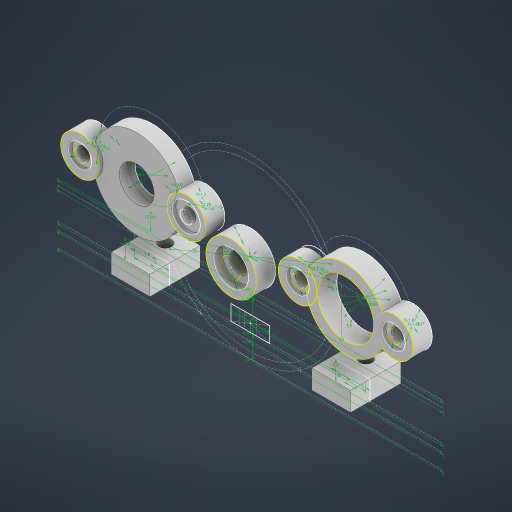
# Autodesk Inventor part: Motormount
Saved by Autodesk Inventor 2023.5 (Build 275446000, 446)
## iProperties
Created: 2024-12-07
Part Number: Motormount
Material: 一般
Document SubType Name: Modeling
Designer: IshiiLabHonda
Density: 1 g/cm^3
Appearance: 既定
Author: IshiiLabHonda
Autodesk Inventor part; units mm, degrees
ref_plane "YZ Plane" through (0, 0, 0) normal (1, 0, 0) x (0, 1, 0)
ref_plane "XZ Plane" through (0, 0, 0) normal (0, 1, 0) x (-1, 0, 0)
ref_plane "XY Plane" through (0, 0, 0) normal (0, 0, 1) x (1, 0, 0)
sketch "blueprint" plane through (0, 0, 0) normal (0, 0, 1) x (1, 0, 0)
  line L0 (0, 0) -> (0, 1) construction
  line L1 (0, 0) -> (1, 0) construction
  circle A0 centre (0, 0) radius 1.25
  circle A1 centre (0, 0) radius 11.5 construction
  line L2 (-25, -11.5) -> (25, -11.5) construction
  line L3 (-25, -9.5) -> (25, -9.5) construction
  line L4 (-25, -8.5) -> (25, -8.5) construction
  line L5 (-25, -4.5) -> (25, -4.5) construction
  circle A2 centre (0, 0) radius 10.65 construction
  circle A3 centre (-12.6949, 2.8) radius 2.25
  circle A4 centre (14.8381, 2.8) radius 4.35 construction
  circle A5 centre (14.8381, 2.8) radius 3.6 construction
  line L6 (-25, -3.7) -> (25, -3.7) construction
  circle A6 centre (-12.6949, 2.8) radius 4.26 construction
  circle A7 centre (-19.5799, 2.8) radius 0.625 construction
  circle A8 centre (-5.8099, 2.8) radius 0.625 construction
  circle A9 centre (-12.6949, 2.8) radius 6.885 construction
  circle A10 centre (-19.5799, 2.8) radius 1.825 construction
  circle A11 centre (-5.8099, 2.8) radius 1.825 construction
  circle A12 centre (14.8381, 2.8) radius 5.1
  circle A13 centre (14.8381, 2.8) radius 6.225 construction
  circle A14 centre (21.0631, 2.8) radius 0.625 construction
  circle A15 centre (8.6131, 2.8) radius 0.625 construction
  circle A16 centre (21.0631, 2.8) radius 1.825 construction
  circle A17 centre (-19.5799, 2.8) radius 0.8
  circle A18 centre (-5.8099, 2.8) radius 0.8
  circle A19 centre (21.0631, 2.8) radius 0.8
  circle A20 centre (-19.5799, 2.8) radius 2.5
  circle A21 centre (-5.8099, 2.8) radius 2.5
  circle A22 centre (21.0631, 2.8) radius 2.5
  circle A23 centre (14.8381, 2.8) radius 3.65
  circle A24 centre (0, 0) radius 3.25
  line L7 (-15, -4.5) -> (-15, -8.5) construction
  line L8 (15, -4.5) -> (15, -8.5) construction
  line L9 (-10.5, -8.5) -> (-10.5, -6)
  line L10 (-15.5, -8.5) -> (-15.5, -6)
  line L11 (-15.5, -6) -> (-10.5, -6)
  line L12 (-13, -6) -> (-13, -8.5)
  line L13 (-13.8, -6) -> (-13.8, -8.5)
  line L14 (-12.2, -6) -> (-12.2, -8.5)
  line L15 (10.5, -8.5) -> (10.5, -6)
  line L16 (15.5, -8.5) -> (15.5, -6)
  line L17 (15.5, -6) -> (10.5, -6)
  line L18 (13, -6) -> (13, -8.5)
  line L19 (13.8, -6) -> (13.8, -8.5)
  line L20 (12.2, -6) -> (12.2, -8.5)
  line L21 (-15.5, -8.5) -> (-10.5, -8.5)
  line L22 (10.5, -8.5) -> (15.5, -8.5)
  circle A25 centre (8.6131, 2.8) radius 1.825 construction
  line L23 (-12.6949, 2.8) -> (-19.5799, 2.8) construction
  line L24 (-12.6949, 2.8) -> (-5.8099, 2.8) construction
  line L25 (14.8381, 2.8) -> (8.6131, 2.8) construction
  circle A26 centre (-12.6949, 2.8) radius 5.76
  line L26 (-2.5, -6.5) -> (2.5, -6.5)
  line L27 (2.5, -6.5) -> (2.5, -8.5)
  line L28 (2.5, -8.5) -> (-2.5, -8.5)
  line L29 (-2.5, -8.5) -> (-2.5, -6.5)
  line L30 (-2.5, -6.5) -> (2.5, -8.5) construction
  line L31 (2.5, -6.5) -> (-2.5, -8.5) construction
  line L32 (0, -6.5) -> (0, -8.5) construction
  line L33 (-0.8, -6.5) -> (-0.8, -8.5) construction
  line L34 (0.8, -6.5) -> (0.8, -8.5) construction
  circle A27 centre (8.6131, 2.8) radius 0.8
  circle A28 centre (8.6131, 2.8) radius 2.5
  line L35 (21.0631, 2.8) -> (14.8381, 2.8) construction
  point P0 (19.5378, 0.8193)
  point P1 (19.5378, 4.7807)
  point P2 (0, -8.5)
  point P3 (-6.4807, -9.5)
  point P4 (6.4807, -9.5)
  point P5 (0, -7.5)
  point P6 (-18.0929, 0.7903)
  point P7 (-7.2969, 0.7903)
  point P8 (-7.2969, 4.8097)
  point P9 (-18.0929, 4.8097)
  dimension "d0" = 1
  dimension "d1" = 1
  dimension "d2" = 2.5
  dimension "d3" = 23
  dimension "d4" = 50
  dimension "d5" = 50
  dimension "d6" = 2
  dimension "d7" = 50
  dimension "d9" = 1
  dimension "d10" = 50
  dimension "d12" = 4
  dimension "d13" = 21.3
  dimension "d14" = 4.5
  dimension "d15" = 8.7
  dimension "d17" = 0.1
  dimension "d18" = 0.1
  dimension "d20" = 7.2
  dimension "d21" = 50
  dimension "d22" = 0.8
  dimension "d23" = 8.52
  dimension "d26" = 1.25
  dimension "d27" = 1.25
  dimension "d28" = 1.2
  dimension "d29" = 1.2
  dimension "d31" = 1.5
  dimension "d32" = 1.25
  dimension "d33" = 1.25
  dimension "d34" = 1.2
  dimension "d37" = 0.5
  dimension "d40" = 1.6
  dimension "d41" = 1.6
  dimension "d43" = 1.6
  dimension "d48" = 7.3
  dimension "d49" = 2
  dimension "d56" = 30
  dimension "d90" = 2.5
  dimension "d92" = 5
  dimension "d93" = 1.6
  dimension "d104" = 1.2
  dimension "d105" = 5
  dimension "d106" = 1.6
  dimension "d107" = 2.5
  dimension "d129" = 5
  dimension "d130" = 5
  dimension "d132" = 5
  dimension "d155" = 26
  dimension "d158" = 1.5
  dimension "d160" = 0.5
  dimension "d161" = 180
  dimension "d166" = 1.6
  dimension "d167" = 5
  dimension "d168" = 2
  dimension "d178" = 1.6
  dimension "d179" = 5
  dimension "d180" = 180
  dimension "d181" = 6.5
  dimension "d187" = 2.24
  constraints: 70 end point, 29 centre point, 24 coincident, 17 point on line, 10 parallel, 8 midpoint, 7 vertical, 6 point on circle, 5 symmetric about line, 4 perpendicular, 3 horizontal, 1 tangent, 18 other
  measures "d0" distance of L0.start L0.end
  measures "d1" distance of L0.start L1.end
  measures "d2" diameter of A0
  measures "d3" diameter of A1
  measures "d4" distance of L2.start L2.end
  measures "d5" distance of L3.start L3.end
  measures "d6" distance between parallel lines of L2 L3
  measures "d7" distance of point (-25, -8.5) point (25, -8.5)
  measures "d10" distance of L5.start L5.end
  measures "d13" diameter of A2
  measures "d14" diameter of A3
  measures "d15" diameter of A4
  measures "d20" diameter of A5
  measures "d21" distance of L6.start L6.end
  measures "d22" distance between parallel lines of L5 L6
  measures "d23" diameter of A6
  measures "d26" diameter of A8
  measures "d27" diameter of A7
  measures "d28" radial gap between concentric circles of A10 A7
  measures "d29" radial gap between concentric circles of A11 A8
  measures "d31" radial gap between concentric circles of A12 A5
  measures "d32" diameter of A14
  measures "d33" diameter of A15
  measures "d34" radial gap between concentric circles of A14 A16
  measures "d40" diameter of A17
  measures "d41" diameter of A18
  measures "d43" diameter of A19
  measures "d48" diameter of A23
  measures "d49" radial gap between concentric circles of A24 A0
  measures "d56" distance between parallel lines of L8 L7
  measures "d90" distance of L10.start L10.end
  measures "d92" distance between parallel lines of L9 L10
  measures "d93" distance between parallel lines of L14 L13
  measures "d104" radial gap between concentric circles of A25 A15
  measures "d105" distance between parallel lines of L16 L15
  measures "d106" distance between parallel lines of L19 L20
  measures "d107" distance of L15.start L15.end
  measures "d129" diameter of A20
  measures "d130" diameter of A21
  measures "d132" diameter of A22
  measures "d155" distance between parallel lines of L18 L12
  measures "d158" radial gap between concentric circles of A26 A6
  measures "d161" angle of L24 L23
  measures "d166" distance between parallel lines of L33 L34
  measures "d167" distance between parallel lines of L27 L29
  measures "d168" distance between parallel lines of L26 L28
  measures "d178" diameter of A27
  measures "d179" diameter of A28
  measures "d180" angle of L25 L35
  measures "d181" distance between parallel lines of L6 L25
  measures "d187" distance edge to line of A6 L6
extrude "押し出し18" add sketch "blueprint" along normal blind 2.5 contours A12 A22 | A12 A22 | A22 A12 A28 | A28 A12 | A18 | A20 A26 | A26 A20 | A26 A21 | A21 A26 | A24 | L21 L14 L11 L9 | L21 L12 L11 L14 | L21 L13 L11 L12 | L21 L10 L11 L13 | L15 L17 L20 L22 | L20 L17 L18 L22 | L18 L17 L19 L22 | L19 L17 L16 L22 picked at (10.2084, 3.3257)
extrude "押し出し19" add sketch "blueprint" against normal blind 4 contours L21 L14 L11 L9 | L21 L12 L11 L14 | L21 L13 L11 L12 | L21 L10 L11 L13 | L15 L17 L20 L22 | L20 L17 L18 L22 | L18 L17 L19 L22 | L19 L17 L16 L22
ref_plane "作業平面1" through (-15.5, -6, 2.5) normal (0, 1, 0) x (1, 0, 0)
sketch "スケッチ2" plane through (-15.5, -6, 2.5) normal (0, 1, 0) x (1, 0, 0)
  line L0 (26, 6.5) -> (26, 0) projected
  line L1 (31, 0) -> (26, 0) projected
  line L2 (31, 6.5) -> (31, 0) projected
  line L3 (26, 6.5) -> (31, 6.5) projected
  line L4 (0, 6.5) -> (0, 0) projected
  line L5 (5, 0) -> (0, 0) projected
  line L6 (5, 0) -> (5, 6.5) projected
  line L7 (0, 6.5) -> (5, 6.5) projected
  line L8 (0, 2.5) -> (5, 2.5) projected
  line L9 (31, 2.5) -> (26, 2.5) projected
  line L10 (0, 6.5) -> (0, 0) projected
  line L11 (5, 2.5) -> (0, 6.5) construction
  line L12 (5, 6.5) -> (5, 0) projected
  line L13 (5, 6.5) -> (0, 2.5) construction
  line L14 (31, 0) -> (31, 6.5) projected
  line L15 (26, 2.5) -> (31, 6.5) construction
  line L16 (26, 6.5) -> (26, 0) projected
  line L17 (31, 2.5) -> (26, 6.5) construction
  circle A0 centre (2.5, 4.5) radius 0.8
  circle A1 centre (28.5, 4.5) radius 0.8
  point P0 (15.5, 2.5)
  dimension "d141" = 1.6
  dimension "d142" = 1.6
  constraints: 8 end point, 2 centre point, 2 midpoint
  measures "d141" diameter of A0
  measures "d142" diameter of A1
extrude "押し出し20" cut sketch "スケッチ2" against normal blind 4 contours A0 | A1
ref_plane "作業平面2" through (0, 0, 2.5) normal (0, 0, 1) x (1, 0, 0)
sketch "スケッチ3" plane through (0, 0, 2.5) normal (0, 0, 1) x (1, 0, 0)
  circle A0 centre (-5.8099, 2.8) radius 2.5 projected
  circle A1 centre (-19.5799, 2.8) radius 2.5 projected
  circle A2 centre (-19.5799, 2.8) radius 0.8 projected
  arc A3 (19.5378, 4.7807) -> (19.5378, 0.8193) centre (14.8381, 2.8) ccw projected
  arc A4 (19.5378, 0.8193) -> (19.5378, 4.7807) centre (21.0631, 2.8) ccw projected
  circle A5 centre (21.0631, 2.8) radius 0.8 projected
  circle A6 centre (14.8381, 2.8) radius 3.65 projected
  circle A7 centre (0, 0) radius 3.25 projected
  circle A8 centre (0, 0) radius 1.25 projected
  circle A9 centre (-19.5799, 2.8) radius 1.5
  circle A10 centre (21.0631, 2.8) radius 0.8 projected
  circle A11 centre (21.0631, 2.8) radius 1.5
  circle A12 centre (0, 0) radius 2.25
  circle A13 centre (-5.8099, 2.8) radius 0.8 projected
  circle A14 centre (-5.8099, 2.8) radius 1.825 construction
  circle A15 centre (-5.8099, 2.8) radius 0.8
  circle A16 centre (-5.8099, 2.8) radius 1.825
  circle A17 centre (8.6131, 2.8) radius 0.8 projected
  circle A18 centre (8.6131, 2.8) radius 2.5 projected
  circle A19 centre (8.6131, 2.8) radius 1.5
  point P0 (10.1385, 4.7807)
  point P1 (10.1385, 0.8193)
  dimension "d146" = 3
  dimension "d148" = 3
  dimension "d150" = 4.5
  dimension "d182" = 3
  constraints: 6 centre point, 6 coincident, 2 concentric
  measures "d146" diameter of A9
  measures "d148" diameter of A11
  measures "d150" diameter of A12
  measures "d182" diameter of A19
extrude "押し出し21" cut sketch "スケッチ3" against normal blind 1.1 contours A12
extrude "押し出し22" cut sketch "スケッチ3" against normal blind 0.5 contours A9 | A11
extrude "押し出し23" cut sketch "スケッチ3" against normal blind 10 contours A13
extrude "押し出し24" cut sketch "スケッチ3" against normal blind 0.5 contours A16
extrude "押し出し28" add sketch "blueprint" along normal blind 2 contours A20 A26 A21
extrude "押し出し29" add sketch "スケッチ3" against normal blind 2 contours A3 A19 A18 | A3 A19 picked at (9.1857, 0.7245) picked at (9.6285, 2.278)
extrude "押し出し30" cut sketch "スケッチ3" against normal blind 0.5 contours A19 A3 | A3 A19
equation "\"d5\" = d4"
equation "\"d7\" = d4"
equation "\"d10\" = d4"
